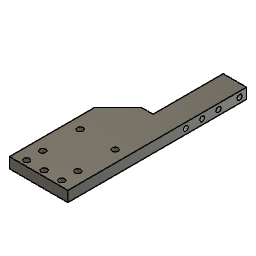
XYConnectorPlate v11 (Autodesk Fusion 360 design; units mm, degrees)
Autodesk Fusion 360 part; units mm, degrees
sketch "Sketch1" plane through (0, 0, 0) normal (0, 1, 0) x (1, 0, 0)
  line L0 (0, 0) -> (50, 0)
  line L1 (50, 0) -> (50, 152.93)
  line L2 (50, 152.93) -> (30, 152.93)
  line L3 (30, 152.93) -> (30, 92.93)
  line L4 (0, 0) -> (0, 72.93)
  line L5 (30, 92.93) -> (20, 92.93)
  line L6 (20, 92.93) -> (0, 72.93)
  circle A0 centre (10, 4.76) radius 2.5
  circle A1 centre (25, 4.76) radius 2.5
  circle A2 centre (40, 4.76) radius 2.5
  line L7 (10, 18.55) -> (40, 18.55) construction
  line L8 (40, 18.55) -> (40, 50.55) construction
  line L9 (40, 50.55) -> (10, 50.55) construction
  line L10 (10, 50.55) -> (10, 18.55) construction
  circle A3 centre (10, 50.55) radius 2.5
  circle A4 centre (40, 50.55) radius 2.5
  circle A5 centre (10, 18.55) radius 2.5
  circle A6 centre (40, 18.55) radius 2.5
  point P0 (10, 50.55)
  dimension "d1" = 50
  dimension "d2" = 152.93
  dimension "d3" = 20
  dimension "d4" = 60
  dimension "d5" = 72.93
  dimension "d6" = 10
  dimension "d16" = 5
  dimension "d17" = 5
  dimension "d18" = 5
  dimension "d19" = 4.76
  dimension "d20" = 10
  dimension "d21" = 4.76
  dimension "d22" = 25
  dimension "d23" = 4.76
  dimension "d24" = 40
  dimension "d33" = 5
  dimension "d34" = 5
  dimension "d35" = 5
  dimension "d36" = 5
  dimension "d37" = 30
  dimension "d38" = 32
  dimension "d39" = 10
  dimension "d40" = 18.55
  constraint coincident L0.start L4.start
  constraint horizontal L0
  constraint perpendicular L0 L1
  constraint perpendicular L1 L2
  constraint perpendicular L2 L3
  constraint perpendicular L0 L4
  constraint perpendicular L3 L5
  constraint horizontal L7
  constraint vertical L8
  constraint horizontal L9
  constraint vertical L10
  constraint coincident P0 L9.end
  constraint coincident L8.end L9.start
  constraint coincident L7.start L10.end
  constraint coincident L7.end L8.start
  measures "d1" distance of L0.start L0.end
  measures "d2" distance of L0.end L1.end
  measures "d3" distance of L1.end L2.end
  measures "d4" distance of L2.end L3.end
  measures "d5" distance of L0.start L4.end
  measures "d6" distance of L3.end L5.end
  measures "d16" diameter of A0
  measures "d17" diameter of A1
  measures "d18" diameter of A2
  measures "d19" distance of L0 A0.centre
  measures "d20" distance of L4 A0.centre
  measures "d21" distance of L0 A1.centre
  measures "d22" distance of L4 A1.centre
  measures "d23" distance of L0 A2.centre
  measures "d24" distance of L4 A2.centre
  measures "d33" diameter of A3
  measures "d34" diameter of A4
  measures "d35" diameter of A5
  measures "d36" diameter of A6
  measures "d37" distance of L8 L10
  measures "d38" distance of L7 L9
  measures "d39" distance of L4 L10
  measures "d40" distance of L0 L7
extrude "Extrude3" add sketch "Sketch1" along normal blind 9
sketch "Sketch4" plane through (30, 0, 0) normal (-1, 0, 0) x (0, 0, 1)
  line L0 (-152.93, 0) -> (-92.93, 0)
  line L1 (-92.93, 0) -> (-92.93, 9)
  line L2 (-92.93, 9) -> (-152.93, 9)
  line L3 (-152.93, 9) -> (-152.93, 0)
  line L4 (-152.93, 4.5) -> (-95, 4.5) construction
  line L5 (-100.93, 9) -> (-100.93, 0) construction
  line L6 (-114.93, 9) -> (-114.93, 0) construction
  line L7 (-128.93, 9) -> (-128.93, 0) construction
  line L8 (-146.93, 9) -> (-146.93, 0) construction
  circle A0 centre (-146.93, 4.5) radius 2.1
  circle A1 centre (-128.93, 4.5) radius 2.1
  circle A2 centre (-114.93, 4.5) radius 2
  circle A3 centre (-100.93, 4.5) radius 2.1
  dimension "d45" = 100.93
  dimension "d46" = 114.93
  dimension "d47" = 128.93
  dimension "d48" = 146.93
  dimension "d49" = 4.2
  dimension "d50" = 4.2
  dimension "d51" = 4
  dimension "d52" = 4.2
  constraint midpoint L3 L4.start
  constraint perpendicular L1 L4
  constraint coincident L2 L5.start
  constraint coincident L0 L5.end
  constraint perpendicular L0 L5
  constraint coincident L2 L6.start
  constraint coincident L0 L6.end
  constraint perpendicular L4 L6
  constraint coincident L2 L7.start
  constraint perpendicular L4 L7
  constraint coincident L2 L8.start
  constraint coincident L0 L8.end
  constraint perpendicular L0 L8
  constraint midpoint L8 A0.centre
  constraint midpoint L7 A1.centre
  constraint midpoint L6 A2.centre
  constraint midpoint L5 A3.centre
  measures "d45" distance of L5 origin
  measures "d46" distance of L6 origin
  measures "d47" distance of L7 origin
  measures "d48" distance of L8 origin
  measures "d49" diameter of A0
  measures "d50" diameter of A1
  measures "d51" diameter of A2
  measures "d52" diameter of A3
hole "Hole2" at (30, 4.5, -146.93) direction (1, 0, 0) diameter 4.2 depth 20 tip angle 118
hole "Hole3" at (30, 4.5, -128.93) direction (1, 0, 0) diameter 4.2 end through all
hole "Hole4" at (30, 4.5, -114.93) direction (1, 0, 0) diameter 4 depth 20 tip angle 118
hole "Hole5" at (30, 4.5, -100.93) direction (1, 0, 0) diameter 4.2 depth 20 tip angle 118
